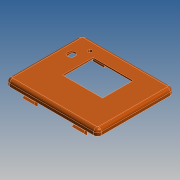
# Autodesk Inventor part: A2_TopCase
Saved by Autodesk Inventor 2020.2 (Build 242310000, 310)
## iProperties
Created: 2021-08-29
Part Number: A2_TopCase
Material: Plastique ABS
Document SubType Name: Modeling
Designer: Samy Francelet
Density: 1.06 g/cm^3
Appearance: Lisse - Orange clair
Author: Samy Francelet
Autodesk Inventor part; units mm, degrees
ref_plane "YZ Plane" through (0, 0, 0) normal (1, 0, 0) x (0, 1, 0)
ref_plane "XZ Plane" through (0, 0, 0) normal (0, 1, 0) x (-1, 0, 0)
ref_plane "XY Plane" through (0, 0, 0) normal (0, 0, 1) x (1, 0, 0)
sketch "Esquisse2" plane through (0, 0, 0) normal (0, 0, 1) x (1, 0, 0)
  line L0 (-85.4497, 0) -> (85.4497, 0) construction
  line L1 (0, -71.4497) -> (0, 71.4497) construction
  line L2 (-55, -50) -> (55, -50)
  line L3 (60, -45) -> (60, 45)
  line L4 (55, 50) -> (-55, 50)
  line L5 (-60, 45) -> (-60, -45)
  line L6 (-60, -50) -> (60, 50) construction
  line L7 (60, -50) -> (-60, 50) construction
  arc A0 (-55, 50) -> (-60, 45) centre (-55, 45) ccw
  arc A1 (-60, -45) -> (-55, -50) centre (-55, -45) ccw
  arc A2 (55, -50) -> (60, -45) centre (55, -45) ccw
  arc A3 (60, 45) -> (55, 50) centre (55, 45) ccw
  point P0 (0, 0)
  dimension "d0" = 120
  dimension "d1" = 100
  dimension "d2" = 5
  constraints: 12 end point, 8 point on circle, 8 point on line, 8 tangent, 4 centre point, 3 equal radius, 2 midpoint, 2 parallel, 1 horizontal, 1 perpendicular
  measures "d0" distance of L7.end L6.end
  measures "d1" distance of L6.end L7.start
  measures "d2" radius of A0
extrude "Extrusion1" add sketch "Esquisse2" along normal blind 8
fillet "Congé1" radius 4 8 edges at (58.5355, -48.5355, 8) (60, 0, 8) (58.5355, 48.5355, 8) (0, 50, 8) (-58.5355, 48.5355, 8) (-60, 0, 8) (-58.5355, -48.5355, 8) (0, -50, 8)
sketch "Esquisse3" plane through (0, 0, 8) normal (0, 0, 1) x (1, 0, 0)
  line L0 (-84, 0) -> (84, 0) construction
  line L1 (0, -70) -> (0, 70) construction
  line L2 (55, 50) -> (-55, 50) construction
  line L3 (-60, 45) -> (-60, -45) construction
  line L4 (-60, 50) -> (-26, 50) construction
  line L5 (-26, 50) -> (-26, 30) construction
  line L6 (-26, 30) -> (-60, 30) construction
  line L7 (-60, 30) -> (-60, 50) construction
  line L8 (-26, 30) -> (26.5, 30)
  line L9 (26.5, 30) -> (26.5, -10)
  line L10 (26.5, -10) -> (-26, -10)
  line L11 (-26, -10) -> (-26, 30)
  point P0 (0, 0)
  dimension "d6" = 34
  dimension "d7" = 20
  dimension "d8" = 52.5
  dimension "d9" = 40
  constraints: 16 end point, 4 parallel, 2 collinear, 2 horizontal, 2 perpendicular
  measures "d6" distance of L5.end L6.end
  measures "d7" distance of L4.end L5.end
  measures "d8" distance of L9.end L10.end
  measures "d9" distance of L8.end L9.end
extrude "Extrusion2" cut sketch "Esquisse3" against normal through all
sketch "Esquisse4" plane through (0, 0, 0) normal (0, 0, -1) x (-1, 0, 0)
  line L0 (0, -70) -> (0, 70) construction
  line L1 (84, 0) -> (-84, 0) construction
  line L2 (-50.5, -42.5) -> (50.5, -42.5)
  line L3 (52.5, -40.5) -> (52.5, 40.5)
  line L4 (50.5, 42.5) -> (-50.5, 42.5)
  line L5 (-52.5, 40.5) -> (-52.5, -40.5)
  line L6 (-52.5, -42.5) -> (52.5, 42.5) construction
  line L7 (52.5, -42.5) -> (-52.5, 42.5) construction
  arc A0 (-50.5, 42.5) -> (-52.5, 40.5) centre (-50.5, 40.5) ccw
  arc A1 (-52.5, -40.5) -> (-50.5, -42.5) centre (-50.5, -40.5) ccw
  arc A2 (50.5, -42.5) -> (52.5, -40.5) centre (50.5, -40.5) ccw
  arc A3 (52.5, 40.5) -> (50.5, 42.5) centre (50.5, 40.5) ccw
  line L8 (-26.5, -10) -> (-26.5, 30) construction
  line L9 (-26.5, 30) -> (26, 30) construction
  line L10 (26, 30) -> (26, -10) construction
  line L11 (26, -10) -> (-26.5, -10) construction
  arc A4 (55, -50) -> (60, -45) centre (55, -45) ccw construction
  line L12 (60, 45) -> (60, -45) construction
  arc A5 (60, 45) -> (55, 50) centre (55, 45) ccw construction
  line L13 (-55, 50) -> (55, 50) construction
  arc A6 (-55, 50) -> (-60, 45) centre (-55, 45) ccw construction
  line L14 (-60, -45) -> (-60, 45) construction
  arc A7 (-60, -45) -> (-55, -50) centre (-55, -45) ccw construction
  line L15 (55, -50) -> (-55, -50) construction
  line L16 (60, 45) -> (60, -45) construction
  line L17 (-55, 50) -> (55, 50) construction
  point P0 (0, 0)
  dimension "d12" = 105
  dimension "d13" = 85
  dimension "d14" = 2
  constraints: 12 end point, 8 point on circle, 8 point on line, 8 tangent, 4 centre point, 3 equal radius, 2 midpoint, 2 parallel, 1 horizontal, 1 perpendicular
  measures "d12" distance of L7.end L6.end
  measures "d13" distance of L6.end L7.start
  measures "d14" radius of A0
extrude "Extrusion3" cut sketch "Esquisse4" against normal blind 6
sketch "Esquisse5" plane through (0, 0, 0) normal (0, 0, -1) x (-1, 0, 0)
  line L0 (0, -70) -> (0, 70) construction
  line L1 (84, 0) -> (-84, 0) construction
  line L2 (-52.5, -40.5) -> (-52.5, 40.5) construction
  arc A0 (-50.5, 42.5) -> (-52.5, 40.5) centre (-50.5, 40.5) ccw construction
  line L3 (-50.5, 42.5) -> (50.5, 42.5) construction
  arc A1 (52.5, 40.5) -> (50.5, 42.5) centre (50.5, 40.5) ccw construction
  line L4 (52.5, 40.5) -> (52.5, -40.5) construction
  arc A2 (50.5, -42.5) -> (52.5, -40.5) centre (50.5, -40.5) ccw construction
  line L5 (50.5, -42.5) -> (-50.5, -42.5) construction
  arc A3 (-52.5, -40.5) -> (-50.5, -42.5) centre (-50.5, -40.5) ccw construction
  arc A4 (55, -50) -> (60, -45) centre (55, -45) ccw construction
  line L6 (60, 45) -> (60, -45) construction
  arc A5 (60, 45) -> (55, 50) centre (55, 45) ccw construction
  line L7 (-55, 50) -> (55, 50) construction
  arc A6 (-55, 50) -> (-60, 45) centre (-55, 45) ccw construction
  line L8 (-60, -45) -> (-60, 45) construction
  arc A7 (-60, -45) -> (-55, -50) centre (-55, -45) ccw construction
  line L9 (55, -50) -> (-55, -50) construction
  line L10 (-60, 50) -> (-40, 50) construction
  line L11 (-40, 50) -> (-40, 43.5) construction
  line L12 (-40, 43.5) -> (-60, 43.5) construction
  line L13 (-60, 43.5) -> (-60, 50) construction
  line L14 (-60, -45) -> (-60, 45) construction
  line L15 (-55, 50) -> (55, 50) construction
  line L16 (-40, 43.5) -> (-25, 43.5)
  line L17 (-25, 43.5) -> (-25, 46.5)
  line L18 (-25, 46.5) -> (-40, 46.5)
  line L19 (-40, 46.5) -> (-40, 43.5)
  point P0 (0, 0)
  dimension "d17" = 20
  dimension "d18" = 6.5
  dimension "d19" = 15
  dimension "d20" = 3
  constraints: 16 end point, 4 parallel, 2 collinear, 2 horizontal, 2 perpendicular
  measures "d17" distance of L11.end L12.end
  measures "d18" distance of L10.end L11.end
  measures "d19" distance of L18.end L17.end
  measures "d20" distance of L17.end L16.end
extrude "Extrusion4" add sketch "Esquisse5" along normal blind 10
sketch "Esquisse6" plane through (25, 46.5, 0) normal (0, 1, 0) x (1, 0, 0)
  line L0 (15, 0) -> (0, 0) construction
  line L1 (15, 0) -> (15, 10) construction
  line L2 (0, 10) -> (15, 10) construction
  line L3 (0, 0) -> (0, 10) construction
  line L4 (0, 10) -> (15, 10)
  line L5 (15, 10) -> (15, 4)
  line L6 (15, 4) -> (0, 4)
  line L7 (0, 4) -> (0, 10)
  point P0 (-25, 0)
  dimension "d23" = 6
  constraints: 8 end point, 2 parallel, 1 horizontal, 1 perpendicular, 1 point on line
  measures "d23" distance of L4.end L5.end
extrude "Extrusion5" add sketch "Esquisse6" along normal blind 2
mirror "Symétrie1" about plane through (0, 0, 0) normal (1, 0, 0) of "Extrusion4", "Extrusion5"
mirror "Symétrie2" about plane through (0, 0, 0) normal (0, 1, 0) of "Extrusion4", "Extrusion5", "Symétrie1"
chamfer "Chanfrein1" distance 4 angle 45 4 edges at (32.5, -48.5, -10) (-32.5, -48.5, -10) (-32.5, 48.5, -10) (32.5, 48.5, -10)
chamfer "Chanfrein2" distance 2 angle 45 4 edges at (32.5, -48.5, -4) (-32.5, -48.5, -4) (32.5, 48.5, -4) (-32.5, 48.5, -4)
sketch "Esquisse9" plane through (0, 0, 6) normal (0, 0, -1) x (-1, 0, 0)
  line L0 (60, 50) -> (35, 50) construction
  line L1 (35, 50) -> (35, 35) construction
  line L2 (35, 35) -> (60, 35) construction
  line L3 (60, 35) -> (60, 50) construction
  line L4 (25, -43.5) -> (40, -43.5) construction
  line L5 (40, -43.5) -> (40, -46.5) construction
  line L6 (40, -46.5) -> (25, -46.5) construction
  line L7 (25, -46.5) -> (25, -43.5) construction
  line L8 (-40, -43.5) -> (-25, -43.5) construction
  line L9 (-25, -43.5) -> (-25, -46.5) construction
  line L10 (-25, -46.5) -> (-40, -46.5) construction
  line L11 (-40, -46.5) -> (-40, -43.5) construction
  line L12 (40, 43.5) -> (25, 43.5) construction
  line L13 (25, 43.5) -> (25, 46.5) construction
  line L14 (25, 46.5) -> (40, 46.5) construction
  line L15 (40, 46.5) -> (40, 43.5) construction
  line L16 (-25, 43.5) -> (-40, 43.5) construction
  line L17 (-40, 43.5) -> (-40, 46.5) construction
  line L18 (-40, 46.5) -> (-25, 46.5) construction
  line L19 (-25, 46.5) -> (-25, 43.5) construction
  arc A0 (52.5, 40.5) -> (50.5, 42.5) centre (50.5, 40.5) ccw construction
  line L20 (52.5, 40.5) -> (52.5, -40.5) construction
  arc A1 (50.5, -42.5) -> (52.5, -40.5) centre (50.5, -40.5) ccw construction
  line L21 (50.5, -42.5) -> (-50.5, -42.5) construction
  arc A2 (-52.5, -40.5) -> (-50.5, -42.5) centre (-50.5, -40.5) ccw construction
  line L22 (-52.5, -40.5) -> (-52.5, 40.5) construction
  arc A3 (-50.5, 42.5) -> (-52.5, 40.5) centre (-50.5, 40.5) ccw construction
  line L23 (-50.5, 42.5) -> (50.5, 42.5) construction
  arc A4 (55, -50) -> (60, -45) centre (55, -45) ccw construction
  line L24 (60, 45) -> (60, -45) construction
  arc A5 (60, 45) -> (55, 50) centre (55, 45) ccw construction
  line L25 (-55, 50) -> (55, 50) construction
  arc A6 (-55, 50) -> (-60, 45) centre (-55, 45) ccw construction
  line L26 (-60, -45) -> (-60, 45) construction
  arc A7 (-60, -45) -> (-55, -50) centre (-55, -45) ccw construction
  line L27 (55, -50) -> (-55, -50) construction
  line L28 (60, 45) -> (60, -45) construction
  line L29 (-55, 50) -> (55, 50) construction
  circle A8 centre (35, 35) radius 4
  point P0 (0, 0)
  dimension "d47" = 25
  dimension "d48" = 15
  dimension "d49" = 8
  constraints: 8 end point, 2 collinear, 2 parallel, 1 centre point, 1 coincident, 1 horizontal, 1 perpendicular
  measures "d47" distance of L2.end L1.end
  measures "d48" distance of L1.end L0.end
  measures "d49" diameter of A8
extrude "Extrusion7" add sketch "Esquisse9" along normal blind 4
sketch "Esquisse7" plane through (0, 0, 8) normal (0, 0, 1) x (1, 0, 0)
  line L0 (-60, 50) -> (-44, 50) construction
  line L1 (-44, 50) -> (-44, 19.5) construction
  line L2 (-44, 19.5) -> (-60, 19.5) construction
  line L3 (-60, 19.5) -> (-60, 50) construction
  line L4 (55, 50) -> (-55, 50) construction
  line L5 (-60, 45) -> (-60, -45) construction
  circle A0 centre (-44, 19.5) radius 5
  line L6 (-60, 50) -> (-35, 50) construction
  line L7 (-35, 50) -> (-35, 35) construction
  line L8 (-35, 35) -> (-60, 35) construction
  line L9 (-60, 35) -> (-60, 50) construction
  circle A1 centre (-35, 35) radius 2.7
  line L10 (-35, 35) -> (-37.2, 35) construction
  line L11 (-37.2, 36.5652) -> (-37.2, 33.4348)
  line L12 (-32.8, 36.5652) -> (-32.8, 33.4348)
  point P0 (0, 0)
  point P1 (-32.8, 33.4348)
  dimension "d32" = 16
  dimension "d33" = 30.5
  dimension "d34" = 10
  dimension "d37" = 25
  dimension "d38" = 15
  dimension "d39" = 5.4
  dimension "d40" = 2.2
  constraints: 22 end point, 4 collinear, 4 parallel, 2 centre point, 2 coincident, 2 horizontal, 2 perpendicular, 2 point on circle, 2 symmetric about line, 1 midpoint, 1 point on line, 1 vertical
  measures "d32" distance of L1.end L2.end
  measures "d33" distance of L0.end L1.end
  measures "d34" diameter of A0
  measures "d37" distance of L7.end L8.end
  measures "d38" distance of L6.end L7.end
  measures "d39" diameter of A1
  measures "d40" distance of L10.start L10.end
extrude "Extrusion6" cut sketch "Esquisse7" against normal through all contours A0 | L12 A1 L11
